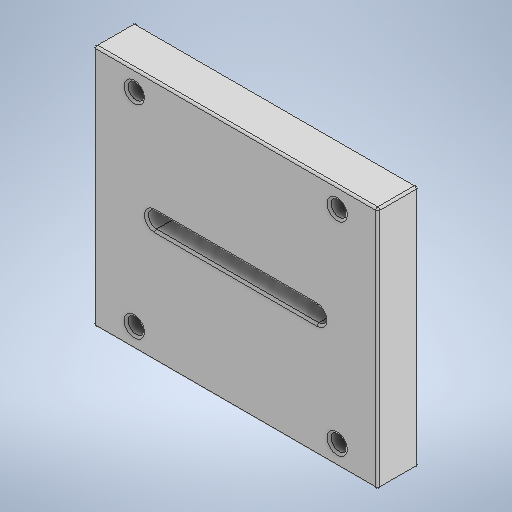
# Autodesk Inventor part: Schiebegewicht Langlochplatte
Saved by Autodesk Inventor 2025 (Build 290162000, 162)
## iProperties
Created: 2026-01-07
Part Number: Schiebegewicht Langlochplatte
Material: Generic
Document SubType Name: Modeling
Designer: ruven
Density: 1 g/cm^3
Appearance: Default
Author: ruven
Autodesk Inventor part; units mm, degrees
ref_plane "YZ Plane" through (0, 0, 0) normal (1, 0, 0) x (0, 1, 0)
ref_plane "XZ Plane" through (0, 0, 0) normal (0, 1, 0) x (-1, 0, 0)
ref_plane "XY Plane" through (0, 0, 0) normal (0, 0, 1) x (1, 0, 0)
sketch "Sketch1" plane through (0, 0, 0) normal (0, 1, 0) x (-1, 0, 0)
  line L0 (-35, -30) -> (35, -30)
  line L1 (35, -30) -> (35, 30)
  line L2 (35, 30) -> (-35, 30)
  line L3 (-35, 30) -> (-35, -30)
  line L4 (-35, -30) -> (35, 30) construction
  line L5 (35, -30) -> (-35, 30) construction
  circle A0 centre (25, 25) radius 2
  circle A1 centre (-25, 25) radius 2
  circle A2 centre (-25, -25) radius 2
  circle A3 centre (25, -25) radius 2
  arc A4 (20, -2) -> (20, 2) centre (20, 0) ccw
  arc A5 (-20, 2) -> (-20, -2) centre (-20, 0) ccw
  line L6 (20, 2) -> (-20, 2)
  line L7 (-20, -2) -> (20, -2)
  point P0 (0, 0)
  dimension "d0" = 70
  dimension "d1" = 60
  dimension "d2" = 4
  dimension "d3" = 4
  dimension "d4" = 4
  dimension "d5" = 4
  dimension "d6" = 10
  dimension "d7" = 10
  dimension "d8" = 10
  dimension "d9" = 10
  dimension "d10" = 5
  dimension "d11" = 5
  dimension "d12" = 5
  dimension "d13" = 5
  dimension "d14" = 40
  dimension "d15" = 20
  dimension "d16" = 4
  dimension "d17" = 4
  constraints: 16 end point, 6 centre point, 4 point on circle, 3 tangent, 2 midpoint, 2 parallel, 1 horizontal, 1 perpendicular
  measures "d0" distance of L1.end L2.end
  measures "d1" distance of L0.end L1.end
  measures "d2" diameter of A3
  measures "d3" diameter of A2
  measures "d4" diameter of A1
  measures "d5" diameter of A0
  measures "d6" distance from line of L1 A0.centre
  measures "d7" distance from line of L1 A3.centre
  measures "d8" distance from line of L3 A2.centre
  measures "d9" distance from line of L3 A1.centre
  measures "d10" distance from line of L2 A1.centre
  measures "d11" distance from line of L2 A0.centre
  measures "d12" distance from line of L0 A3.centre
  measures "d13" distance from line of L0 A2.centre
  measures "d14" distance of A5.centre A4.centre
  measures "d15" distance of point (0, 0) A5.centre
  measures "d16" diameter of A4
  measures "d17" diameter of A5
extrude "Extrusion1" add sketch "Sketch1" along normal blind 10
fillet "Fillet1" radius 0.5 28 edges at (-35, 10, 0) (0, 10, 30) (35, 5, -30) (35, 5, 30) (35, 0, 0) (35, 10, 0) (-35, 0, 0) (-35, 5, 30) (27, 10, -25) (-23, 0, 25) (-23, 10, 25) (0, 0, 30) (0, 10, -30) (0, 0, -30) (-23, 10, -25) (-23, 0, -25) (-35, 5, -30) (-22, 10, 0) (0, 10, -2) (22, 10, 0) (0, 10, 2) (22, 0, 0) (0, 0, 2) (-22, 0, 0) (0, 0, -2) (27, 10, 25) (27, 0, 25) (27, 0, -25)
body "Solid1"
